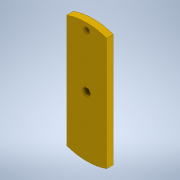
# Autodesk Inventor part: driveForPiston-8-inV03
Saved by Autodesk Inventor 2020.2 (Build 242310000, 310)
## iProperties
Created: 2020-01-13
Part Number: driveForPiston-8-inV03
Material: PET Plastic
Document SubType Name: Modeling
Designer: robst
Density: 1.541 g/cm^3
Appearance: Gold
Author: robst
Autodesk Inventor part; units mm, degrees
ref_plane "YZ Plane" through (0, 0, 0) normal (1, 0, 0) x (0, 1, 0)
ref_plane "XZ Plane" through (0, 0, 0) normal (0, 1, 0) x (-1, 0, 0)
ref_plane "XY Plane" through (0, 0, 0) normal (0, 0, 1) x (1, 0, 0)
sketch "Sketch1" plane through (0, 0, 0) normal (0, 0, 1) x (1, 0, 0)
  circle A0 centre (0, 0) radius 114.3
  line L0 (7.6256, 0) -> (3.8128, -6.604)
  line L1 (3.8128, -6.604) -> (-3.8128, -6.604)
  line L2 (-3.8128, -6.604) -> (-7.6256, 0)
  line L3 (-7.6256, 0) -> (-3.8128, 6.604)
  line L4 (-3.8128, 6.604) -> (3.8128, 6.604)
  line L5 (3.8128, 6.604) -> (7.6256, 0)
  circle A1 centre (0, 101.6) radius 5.2705
  dimension "d0" = 228.6
  dimension "d1" = 13.208
  dimension "d2" = 10.541
  dimension "d5" = 101.6
  constraints: 12 end point, 2 centre point, 2 coincident, 1 horizontal, 13 other
  measures "d0" diameter of A0
  measures "d1" distance between parallel lines of L1 L4
  measures "d2" diameter of A1
  measures "d5" distance of A1.centre point (0, 0)
extrude "Extrusion1" add sketch "Sketch1" along normal mid plane 12.7
sketch "Sketch4" plane through (0, 0, 6.35) normal (0, 0, 1) x (1, 0, 0)
  circle A0 centre (0, 0) radius 114.3 projected
  line L0 (-38.1, 107.7631) -> (-38.1, -107.7631)
  line L1 (38.1, 107.7631) -> (38.1, -107.7631)
  arc A1 (-38.1, 107.7631) -> (-38.1, -107.7631) centre (0, 0) ccw
  arc A2 (38.1, -107.7631) -> (38.1, 107.7631) centre (0, 0) ccw
  dimension "d18" = 38.1
  dimension "d19" = 38.1
  constraints: 8 point on circle, 4 end point, 2 centre point, 2 vertical, 1 coincident
  measures "d18" distance from line of L0 point (0, 0)
  measures "d19" distance from line of L1 point (0, 0)
extrude "Extrusion4" cut sketch "Sketch4" against normal through all contours A0 L1 | L0 A0
sketch "Sketch2" plane through (0, 0, 6.35) normal (0, 0, 1) x (1, 0, 0)
  circle A0 centre (-63.5, 0) radius 25.4
  circle A1 centre (-31.75, -54.9926) radius 25.4
  circle A2 centre (31.75, -54.9926) radius 25.4
  circle A3 centre (63.5, 0) radius 25.4
  circle A4 centre (31.75, 54.9926) radius 25.4
  circle A5 centre (-31.75, 54.9926) radius 25.4
  point P0 (0, 0)
  dimension "d6" = 50.8
  dimension "d7" = 63.5
  dimension "d10" = 360
  constraints: 6 centre point, 13 other
  measures "d6" diameter of A0
  measures "d7" distance of A0.centre point (0, 0)
body "Solid1"
